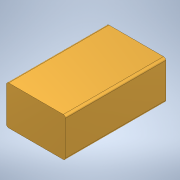
# Autodesk Inventor part: Battery06P
Saved by Autodesk Inventor 2020.2 (Build 242310000, 310)
## iProperties
Created: 2020-03-30
Part Number: Battery06P
Material: 一般
Document SubType Name: Modeling
Designer: aoyama
Mass: 45 g
Surface Area: 49.5147 cm^2
Volume: 21.0638 cm^3
Density: 2.13637 g/cm^3
Appearance: 真鍮 - サテン
Author: aoyama
Autodesk Inventor part; units mm, degrees
ref_plane "YZ Plane" through (0, 0, 0) normal (1, 0, 0) x (0, 1, 0)
ref_plane "XZ Plane" through (0, 0, 0) normal (0, 1, 0) x (-1, 0, 0)
ref_plane "XY Plane" through (0, 0, 0) normal (0, 0, 1) x (1, 0, 0)
sketch "スケッチ1" plane through (0, 0, 0) normal (0, 0, 1) x (1, 0, 0)
  line L0 (0, 0) -> (-26.5, 0)
  line L1 (-26.5, 0) -> (-26.5, 17.5)
  line L2 (-26.5, 17.5) -> (0, 17.5)
  line L3 (0, 17.5) -> (0, 0)
  circle A0 centre (-18.5164, 8.75) radius 3.5
  circle A1 centre (-6.7964, 8.75) radius 3
  dimension "d1" = 26.5
  dimension "d2" = 17.5
  dimension "d3" = 7
  dimension "d4" = 6
  dimension "d5" = 8.75
  dimension "d6" = 8.75
  constraints: 8 end point, 2 centre point, 2 parallel, 1 horizontal, 1 vertical
  measures "d1" distance of L1.end L2.end
  measures "d2" distance of L2.end L0.start
  measures "d3" diameter of A0
  measures "d4" diameter of A1
  measures "d5" distance from line of L2 A0.centre
  measures "d6" distance from line of L2 A1.centre
extrude "押し出し1" add sketch "スケッチ1" along normal blind 45 contours L0 L1 L2 L3 | A0 | A1
extrude "押し出し2" add sketch "スケッチ1" against normal blind 3.5 contours A0 | A1
fillet "フィレット1" radius 1 4 edges at (-26.5, 17.5, 22.5) (-26.5, 0, 22.5) (0, 17.5, 22.5) (0, 0, 22.5)
